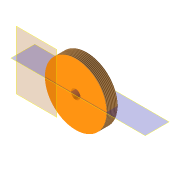
# Autodesk Inventor part: ESP32ParasiteMicroscope_focusknob_v0
Saved by Autodesk Inventor 2022 (Build 260153000, 153)
## iProperties
Created: 2022-02-02
Part Number: ESP32ParasiteMicroscope_focusknob_v0
Material: Generisch
Document SubType Name: Modeling
Designer: diederichbenedict
Density: 1 g/cm^3
Appearance: Orange
Author: diederichbenedict
Autodesk Inventor part; units mm, degrees
ref_plane "YZ Plane" through (0, 0, 0) normal (1, 0, 0) x (0, 1, 0)
ref_plane "XZ Plane" through (0, 0, 0) normal (0, 1, 0) x (-1, 0, 0)
ref_plane "XY Plane" through (0, 0, 0) normal (0, 0, 1) x (1, 0, 0)
ref_plane "Arbeitsebene1" through (0, 0, 0) normal (0, 0, 1) x (1, 0, 0)
sketch "Skizze1" plane through (0, 0, 0) normal (0, 0, 1) x (1, 0, 0)
  spline S0 degree 3 poles (-17.6341, -17.1367) (-21.1223, -14.0447) (-23.6303, -9.8629) (-24.7151, -5.3296) (-25.803, -0.7834) (-25.4545, 4.0955) (-23.7315, 8.441) (-22.4146, 11.7621) (-20.3077, 14.7669) (-17.6341, 17.1367) knots 5.437647 5.437647 5.437647 5.437647 6.048298 6.048298 6.048298 6.66069 6.66069 6.66069 7.128724 7.128724 7.128724 7.128724 projected
  arc A0 (16.0826, -13.4603) -> (16.0826, 13.4603) centre (-2.4439, 0) ccw projected
  circle A1 centre (-2.4439, 0) radius 22.5
  circle A2 centre (-2.4439, 0) radius 3.45
  point P0 (0, 0)
  dimension "d0" = 45
  dimension "d1" = 6.9
  constraints: 2 centre point, 2 coincident
  measures "d0" diameter of A1
  measures "d1" diameter of A2
extrude "Extrusion1" add sketch "Skizze1" against normal blind 8
ref_plane "Arbeitsebene2" through (-41.5374, 0, -15.8898) normal (0, -1, 0) x (1, 0, 0)
sketch "Skizze3" plane through (-2.4439, 0, -8) normal (0, 0, -1) x (-1, 0, 0)
  circle A0 centre (0, 0) radius 3.45 projected
  circle A1 centre (0, 0) radius 20
  point P0 (-2.4439, 0)
  dimension "d20" = 40
  constraints: 1 centre point, 1 coincident
  measures "d20" diameter of A1
extrude "Extrusion2" cut sketch "Skizze3" against normal blind 3 contours A0 | A1
thread "Gewinde1" size "M45x1" class "6g" standard "ANSI Metric M Profile" full length
